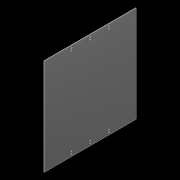
# Autodesk Inventor part: TopV5
Saved by Autodesk Inventor 2022 (Build 260153000, 153)
## iProperties
Created: 2021-10-02
Part Number: TopV5
Material: Steel
Document SubType Name: Sheet Metal
Designer: timmy
Density: 7.85 g/cm^3
Appearance: Smooth - Black
Sheet Metal Rule: Default
Author: timmy
Autodesk Inventor part; units mm, degrees
ref_plane "YZ Plane" through (0, 0, 0) normal (1, 0, 0) x (0, 1, 0)
ref_plane "XZ Plane" through (0, 0, 0) normal (0, 1, 0) x (-1, 0, 0)
ref_plane "XY Plane" through (0, 0, 0) normal (0, 0, 1) x (1, 0, 0)
sketch "Sketch1" plane through (0, 0, 0) normal (1, 0, 0) x (0, 1, 0)
  line L0 (0, 0) -> (533.4, 0)
  line L1 (533.4, 0) -> (533.4, -508)
  line L2 (533.4, -508) -> (0, -508)
  line L3 (0, -508) -> (0, 0)
  dimension "d0" = 533.4
  dimension "d1" = 508
  constraints: 8 end point, 2 parallel, 1 horizontal, 1 perpendicular
  measures "d0" distance of L1.end L2.end
  measures "d1" distance of L0.end L1.end
extrude "Extrusion1" add sketch "Sketch1" along normal blind 1.5875
sketch "Sketch3" plane through (0, 0, 0) normal (-1, 0, 0) x (0, 0, 1)
  line L0 (-508, 0) -> (-508, 533.4) projected
  line L1 (0, 0) -> (-508, 0) projected
  circle A0 centre (-358.14, 12.7) radius 3.302
  circle A1 centre (-358.14, 25.4) radius 3.302
  circle A2 centre (-149.86, 12.7) radius 3.302
  circle A3 centre (-149.86, 25.4) radius 3.302
  circle A4 centre (-254, 12.7) radius 3.302
  circle A5 centre (-254, 25.4) radius 3.302
  circle A6 centre (-358.14, 508) radius 3.302
  circle A7 centre (-358.14, 520.7) radius 3.302
  circle A8 centre (-149.86, 508) radius 3.302
  circle A9 centre (-149.86, 520.7) radius 3.302
  circle A10 centre (-254, 508) radius 3.302
  circle A11 centre (-254, 520.7) radius 3.302
  constraints: 12 centre point
extrude "Extrusion5" cut sketch "Sketch3" against normal up to surface (1.5875 mm away) contours A0 | A1 | A2 | A3 | A4 | A5
sheet face with bend "Face1" sketch "Sketch1" thickness 3.048 toward (1, 0, 0) bend radius 3.048 relief straight relief width 3.048 relief depth 1.524
bend "Bend1"
extrude "Cut1" cut sketch "Sketch3" against normal up to surface (3.048 mm away)
equation "\"d38\" = Thickness"
equation "\"d32\" = Thickness"
equation "\"d33\" = BendRadius"
equation "\"d34\" = BendReliefWidth"
equation "\"d36\" = MinimumRemnant"
equation "\"d35\" = BendReliefDepth"
equation "\"d37\" = TransitionRadius"
equation "\"BendRadius\" = Thickness"
equation "\"BendReliefWidth\" = Thickness"
equation "\"BendReliefDepth\" = 0.5 * Thickness"
equation "\"CornerReliefSize\" = 4 * Thickness"
equation "\"MinimumRemnant\" = 2 * Thickness"
equation "\"TransitionRadius\" = BendRadius"
equation "\"JacobiRadiusSize\" = BendRadius"
equation "\"GapSize\" = Thickness"
equation "\"Thickness\" = 3.048"
body "Solid1"
